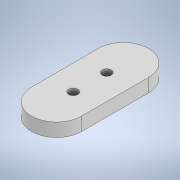
# Autodesk Inventor part: Bottom_Foot
Saved by Autodesk Inventor 2021 (Build 250183000, 183)
## iProperties
Created: 2021-05-04
Part Number: Bottom_Foot
Material: Generic
Document SubType Name: Modeling
Designer: Jorian Brusind
Density: 1 g/cm^3
Appearance: Default
Author: Jorian Brusind
Autodesk Inventor part; units mm, degrees
ref_plane "YZ Plane" through (0, 0, 0) normal (1, 0, 0) x (0, 1, 0)
ref_plane "XZ Plane" through (0, 0, 0) normal (0, 1, 0) x (-1, 0, 0)
ref_plane "XY Plane" through (0, 0, 0) normal (0, 0, 1) x (1, 0, 0)
sketch "Sketch1" plane through (0, 0, 0) normal (0, 1, 0) x (-1, 0, 0)
  line L0 (0, 20) -> (0, -20) construction
  line L1 (-15, 20) -> (-15, -20)
  line L2 (15, -20) -> (15, 20)
  arc A0 (15, 20) -> (-15, 20) centre (0, 20) ccw
  arc A1 (-15, -20) -> (15, -20) centre (0, -20) ccw
  point P0 (0, 0)
  dimension "d0" = 20
  dimension "d1" = 30
  constraints: 8 end point, 4 point on circle, 4 tangent, 2 centre point, 1 midpoint, 1 parallel, 1 vertical
  measures "d0" distance of point (0, 0) L0.end
  measures "d1" diameter of A1
extrude "Extrusion1" add sketch "Sketch1" along normal blind 8
sketch "Sketch2" plane through (0, 0, 0) normal (0, -1, 0) x (1, 0, 0)
  circle A0 centre (0, -10) radius 4.5
  line L0 (15, 20) -> (15, -20) projected
  circle A1 centre (0, 10) radius 4.5
  point P0 (0, 0)
  dimension "d4" = 9
  dimension "d5" = 10
  dimension "d6" = 15
  dimension "d7" = 9
  dimension "d8" = 15
  dimension "d9" = 10
  constraints: 2 centre point
  measures "d4" diameter of A0
  measures "d5" distance of point (0, 0) A0.centre
  measures "d6" distance from line of L0 A0.centre
  measures "d7" diameter of A1
  measures "d8" distance from line of L0 A1.centre
  measures "d9" distance of point (0, 0) A1.centre
extrude "Extrusion2" cut sketch "Sketch2" against normal blind 3
sketch "Sketch3" plane through (0, 3, 10) normal (0, -1, 0) x (1, 0, 0)
  circle A0 centre (0, 0) radius 4.5 projected
  circle A1 centre (0, 0) radius 2.75
  circle A2 centre (0, -20) radius 4.5 projected
  circle A3 centre (0, -20) radius 2.75
  point P0 (0, -10)
  dimension "d12" = 5.5
  dimension "d13" = 5.5
  constraints: 2 centre point, 2 coincident
  measures "d12" diameter of A1
  measures "d13" diameter of A3
extrude "Extrusion3" cut sketch "Sketch3" against normal through all contours A1 | A3
body "Solid1"
